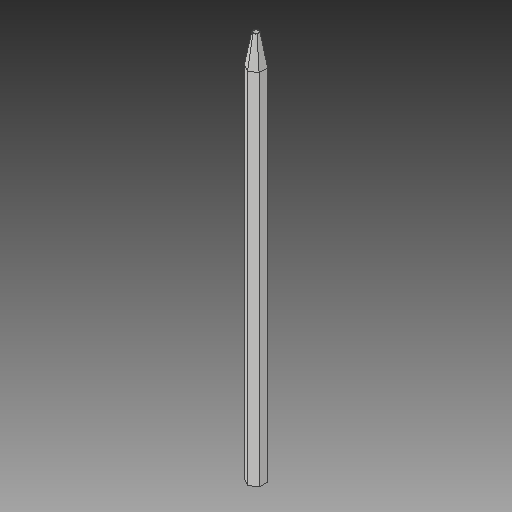
# Autodesk Inventor part: Pencil Shell
Saved by Autodesk Inventor 2017 (Build 210142000, 142)
## iProperties
Created: 2015-08-30
Part Number: Pencil Shell
Material: Generic
Document SubType Name: Modeling
Density: 1 g/cm^3
Appearance: Default
Autodesk Inventor part; units mm, degrees
ref_plane "YZ Plane" through (0, 0, 0) normal (1, 0, 0) x (0, 1, 0)
ref_plane "XZ Plane" through (0, 0, 0) normal (0, 1, 0) x (-1, 0, 0)
sketch "Sketch1" plane through (0, 0, 0) normal (0, 1, 0) x (-1, 0, 0)
  line L0 (2.45, -1.4145) -> (0, -2.829)
  line L1 (0, -2.829) -> (-2.45, -1.4145)
  line L2 (-2.45, -1.4145) -> (-2.45, 1.4145)
  line L3 (-2.45, 1.4145) -> (0, 2.829)
  line L4 (0, 2.829) -> (2.45, 1.4145)
  line L5 (2.45, 1.4145) -> (2.45, -1.4145)
  point P0 (0, 0)
  point P1 (0, 0)
  dimension "d0" = 4.9
  constraints: 12 end point, 1 coincident, 13 other
  measures "d0" distance between parallel lines of L2 L5
extrude "Extrusion1" add sketch "Sketch1" along normal blind 120
ref_plane "Work Plane1" through (0, 130, 0) normal (0, 1, 0) x (1, 0, 0)
sketch "Sketch2" plane through (0, 120, 0) normal (0, 1, 0) x (1, 0, 0)
  line L0 (-2.45, 1.4145) -> (0, 2.829)
  line L1 (0, 2.829) -> (2.45, 1.4145)
  line L2 (2.45, 1.4145) -> (2.45, -1.4145)
  line L3 (2.45, -1.4145) -> (0, -2.829)
  line L4 (0, -2.829) -> (-2.45, -1.4145)
  line L5 (-2.45, -1.4145) -> (-2.45, 1.4145)
  point P0 (0, 0)
  point P1 (0, 0)
  dimension "d4" = 4.9
  constraints: 12 end point, 1 coincident, 13 other
  measures "d4" distance between parallel lines of L2 L5
sketch "Sketch3" plane through (0, 130, 0) normal (0, 1, 0) x (1, 0, 0)
  circle A0 centre (0, 0) radius 1
  dimension "d5" = 2
  constraints: 1 centre point, 1 coincident
  measures "d5" diameter of A0
loft "Loft1" add profiles "Sketch3" section 1 edges at (-1.225, 120, -2.1218) (-2.45, 120, 0) (-1.225, 120, 2.1218) (1.225, 120, 2.1218) (2.45, 120, 0) (1.225, 120, -2.1218)
hole "Hole1" at (0, 130, 0) direction (0, -1, 0) diameter 1.5 end through all
body "Solid1"
